Autodesk Fusion 360 part; units mm, degrees
(part 10 of 20)
  spline S928 degree 3 poles (18.9628, -686.0109) (18.8503, -686.0753) (18.6416, -686.1948) (18.4191, -686.286) (18.3165, -686.3281) knots 0 0 0 0 0.03884 0.072064 0.072064 0.072064 0.072064
  line L317 (18.3165, -686.3281) -> (18.3165, -685.7346)
  spline S929 degree 3 poles (18.3165, -685.7346) (18.4811, -685.6511) (18.8025, -685.4881) (19.081, -685.2595) (19.2169, -685.148) knots 0 0 0 0 0.05519 0.10775 0.10775 0.10775 0.10775
  spline S930 degree 3 poles (19.2169, -685.148) (19.3329, -685.0399) (19.5456, -684.8418) (19.6947, -684.5927) (19.7626, -684.4795) knots 0 0 0 0 0.047275 0.086674 0.086674 0.086674 0.086674
  line L318 (19.7626, -684.4795) -> (20.1582, -684.4795)
  line L319 (20.1582, -684.4795) -> (20.1583, -689.5)
  line L320 (29.2799, -739.4997) -> (29.2798, -735.8776)
  line L321 (29.2798, -735.8776) -> (29.8289, -735.8776)
  line L322 (29.8289, -735.8776) -> (29.8289, -736.3858)
  spline S931 degree 3 poles (29.8289, -736.3858) (29.8908, -736.3012) (30.0157, -736.1307) (30.1931, -736.0157) (30.2825, -735.9577) knots 0 0 0 0 0.031158 0.062835 0.062835 0.062835 0.062835
  spline S932 degree 3 poles (30.2825, -735.9577) (30.3817, -735.9105) (30.5856, -735.8134) (30.8112, -735.8017) (30.9271, -735.7957) knots 0 0 0 0 0.032617 0.067048 0.067048 0.067048 0.067048
  spline S933 degree 3 poles (30.9271, -735.7957) (31.0516, -735.8004) (31.284, -735.8093) (31.491, -735.9141) (31.5871, -735.9628) knots 0 0 0 0 0.036859 0.068796 0.068796 0.068796 0.068796
  spline S934 degree 3 poles (31.5871, -735.9628) (31.6668, -736.0245) (31.8277, -736.1492) (31.9092, -736.3358) (31.9503, -736.4301) knots 0 0 0 0 0.029725 0.060035 0.060035 0.060035 0.060035
  spline S935 degree 3 poles (31.9503, -736.4301) (32.1005, -736.2451) (32.3916, -735.8865) (32.848, -735.8253) (33.069, -735.7957) knots 0 0 0 0 0.068625 0.133023 0.133023 0.133023 0.133023
  spline S936 degree 3 poles (33.069, -735.7957) (33.2341, -735.8041) (33.542, -735.8197) (33.7851, -736.0072) (33.8978, -736.0941) knots 0 0 0 0 0.048244 0.08997 0.08997 0.08997 0.08997
  spline S937 degree 3 poles (33.8978, -736.0941) (33.9821, -736.2164) (34.1715, -736.4913) (34.1819, -736.8269) (34.1877, -737.0132) knots 0 0 0 0 0.043695 0.098195 0.098195 0.098195 0.098195
  line L323 (34.1877, -737.0132) -> (34.1878, -739.4996)
  line L324 (34.1878, -739.4996) -> (33.5773, -739.4996)
  line L325 (33.5773, -739.4996) -> (33.5772, -737.2179)
  spline S938 degree 3 poles (33.5772, -737.2179) (33.5772, -737.1117) (33.5772, -736.9323) (33.5348, -736.7584) (33.5175, -736.6875) knots 0 0 0 0 0.031711 0.053535 0.053535 0.053535 0.053535
  spline S939 degree 3 poles (33.5175, -736.6875) (33.4931, -736.6359) (33.4432, -736.5305) (33.349, -736.4617) (33.3009, -736.4266) knots 0 0 0 0 0.016863 0.034394 0.034394 0.034394 0.034394
  spline S940 degree 3 poles (33.3009, -736.4266) (33.2452, -736.3978) (33.1298, -736.338) (32.9998, -736.3312) (32.9326, -736.3277) knots 0 0 0 0 0.018597 0.038532 0.038532 0.038532 0.038532
  spline S941 degree 3 poles (32.9326, -736.3277) (32.8115, -736.3375) (32.5735, -736.3568) (32.3889, -736.5077) (32.2982, -736.5818) knots 0 0 0 0 0.035532 0.069798 0.069798 0.069798 0.069798
  spline S942 degree 3 poles (32.2982, -736.5818) (32.2249, -736.6885) (32.0578, -736.9317) (32.0501, -737.2286) (32.0459, -737.3953) knots 0 0 0 0 0.038079 0.086792 0.086792 0.086792 0.086792
  line L326 (32.0459, -737.3953) -> (32.0459, -739.4996)
  line L327 (32.0459, -739.4996) -> (31.432, -739.4997)
  line L328 (31.432, -739.4997) -> (31.4319, -737.1463)
  spline S943 degree 3 poles (31.4319, -737.1463) (31.4295, -737.0243) (31.4252, -736.8075) (31.3254, -736.6161) (31.2818, -736.5324) knots 0 0 0 0 0.036008 0.063954 0.063954 0.063954 0.063954
  spline S944 degree 3 poles (31.2818, -736.5324) (31.2196, -736.4728) (31.0834, -736.3424) (30.8937, -736.3329) (30.7907, -736.3278) knots 0 0 0 0 0.025037 0.054812 0.054812 0.054812 0.054812
  spline S945 degree 3 poles (30.7907, -736.3278) (30.706, -736.3335) (30.5365, -736.3448) (30.3865, -736.4244) (30.3115, -736.4642) knots 0 0 0 0 0.025172 0.050327 0.050327 0.050327 0.050327
  spline S946 degree 3 poles (30.3115, -736.4642) (30.2429, -736.5159) (30.1026, -736.6215) (30.0298, -736.7815) (29.9926, -736.8633) knots 0 0 0 0 0.025339 0.051812 0.051812 0.051812 0.051812
  spline S947 degree 3 poles (29.9926, -736.8633) (29.9639, -736.9696) (29.8971, -737.2171) (29.895, -737.4739) (29.8937, -737.6204) knots 0 0 0 0 0.032907 0.076633 0.076633 0.076633 0.076633
  line L329 (29.8937, -737.6204) -> (29.8938, -739.4997)
  line L330 (29.8938, -739.4997) -> (29.2799, -739.4997)
  line L331 (20.1598, -739.4999) -> (19.5459, -739.4999)
  line L332 (19.5459, -739.4999) -> (19.5458, -735.5879)
  spline S948 degree 3 poles (19.5458, -735.5879) (19.4621, -735.6608) (19.2807, -735.8186) (19.0751, -735.9436) (18.9643, -736.0109) knots 0 0 0 0 0.033221 0.072019 0.072019 0.072019 0.072019
  spline S949 degree 3 poles (18.9643, -736.0109) (18.8518, -736.0753) (18.6431, -736.1948) (18.4206, -736.286) (18.318, -736.3281) knots 0 0 0 0 0.03884 0.072064 0.072064 0.072064 0.072064
  line L333 (18.318, -736.3281) -> (18.318, -735.7346)
  spline S950 degree 3 poles (18.318, -735.7346) (18.4826, -735.6511) (18.804, -735.488) (19.0825, -735.2595) (19.2184, -735.148) knots 0 0 0 0 0.05519 0.10775 0.10775 0.10775 0.10775
  spline S951 degree 3 poles (19.2184, -735.148) (19.3344, -735.0399) (19.5471, -734.8418) (19.6962, -734.5927) (19.7641, -734.4795) knots 0 0 0 0 0.047275 0.086674 0.086674 0.086674 0.086674
  line L334 (19.7641, -734.4795) -> (20.1597, -734.4795)
  line L335 (20.1597, -734.4795) -> (20.1598, -739.4999)
  line L336 (28.5502, -789.465) -> (28.5499, -785.8429)
  line L337 (28.5499, -785.8429) -> (29.0991, -785.8429)
  line L338 (29.0991, -785.8429) -> (29.0991, -786.3511)
  spline S952 degree 3 poles (29.0991, -786.3511) (29.161, -786.2665) (29.2859, -786.096) (29.4633, -785.981) (29.5527, -785.923) knots 0 0 0 0 0.031158 0.062835 0.062835 0.062835 0.062835
  spline S953 degree 3 poles (29.5527, -785.923) (29.6519, -785.8758) (29.8557, -785.7786) (30.0814, -785.767) (30.1973, -785.761) knots 0 0 0 0 0.032617 0.067048 0.067048 0.067048 0.067048
  spline S954 degree 3 poles (30.1973, -785.761) (30.3218, -785.7657) (30.5542, -785.7745) (30.7612, -785.8794) (30.8572, -785.928) knots 0 0 0 0 0.036859 0.068796 0.068796 0.068796 0.068796
  spline S955 degree 3 poles (30.8572, -785.928) (30.9369, -785.9898) (31.0979, -786.1144) (31.1794, -786.301) (31.2205, -786.3953) knots 0 0 0 0 0.029725 0.060035 0.060035 0.060035 0.060035
  spline S956 degree 3 poles (31.2205, -786.3953) (31.3707, -786.2103) (31.6618, -785.8517) (32.1182, -785.7905) (32.3392, -785.7608) knots 0 0 0 0 0.068625 0.133023 0.133023 0.133023 0.133023
  spline S957 degree 3 poles (32.3392, -785.7608) (32.5042, -785.7692) (32.8121, -785.7849) (33.0552, -785.9723) (33.168, -786.0592) knots 0 0 0 0 0.048244 0.08997 0.08997 0.08997 0.08997
  spline S958 degree 3 poles (33.168, -786.0592) (33.2523, -786.1815) (33.4417, -786.4564) (33.4522, -786.792) (33.4579, -786.9783) knots 0 0 0 0 0.043695 0.098195 0.098195 0.098195 0.098195
  line L339 (33.4579, -786.9783) -> (33.4581, -789.4647)
  line L340 (33.4581, -789.4647) -> (32.8476, -789.4647)
  line L341 (32.8476, -789.4647) -> (32.8475, -787.183)
  spline S959 degree 3 poles (32.8475, -787.183) (32.8474, -787.0768) (32.8474, -786.8975) (32.805, -786.7235) (32.7877, -786.6526) knots 0 0 0 0 0.031711 0.053535 0.053535 0.053535 0.053535
  spline S960 degree 3 poles (32.7877, -786.6526) (32.7633, -786.601) (32.7134, -786.4956) (32.6192, -786.4268) (32.5711, -786.3918) knots 0 0 0 0 0.016863 0.034394 0.034394 0.034394 0.034394
  spline S961 degree 3 poles (32.5711, -786.3918) (32.5154, -786.3629) (32.4, -786.3032) (32.27, -786.2964) (32.2028, -786.2929) knots 0 0 0 0 0.018597 0.038532 0.038532 0.038532 0.038532
  spline S962 degree 3 poles (32.2028, -786.2929) (32.0816, -786.3027) (31.8437, -786.3219) (31.6591, -786.4729) (31.5684, -786.547) knots 0 0 0 0 0.035532 0.069798 0.069798 0.069798 0.069798
  spline S963 degree 3 poles (31.5684, -786.547) (31.4951, -786.6537) (31.328, -786.8969) (31.3204, -787.1938) (31.3161, -787.3605) knots 0 0 0 0 0.038079 0.086792 0.086792 0.086792 0.086792
  line L342 (31.3161, -787.3605) -> (31.3162, -789.4648)
  line L343 (31.3162, -789.4648) -> (30.7023, -789.4649)
  line L344 (30.7023, -789.4649) -> (30.7022, -787.1115)
  spline S964 degree 3 poles (30.7022, -787.1115) (30.6997, -786.9895) (30.6954, -786.7727) (30.5956, -786.5813) (30.552, -786.4976) knots 0 0 0 0 0.036008 0.063954 0.063954 0.063954 0.063954
  spline S965 degree 3 poles (30.552, -786.4976) (30.4898, -786.4381) (30.3536, -786.3077) (30.1639, -786.2982) (30.0609, -786.293) knots 0 0 0 0 0.025037 0.054812 0.054812 0.054812 0.054812
  spline S966 degree 3 poles (30.0609, -786.293) (29.9761, -786.2987) (29.8067, -786.3101) (29.6567, -786.3897) (29.5817, -786.4295) knots 0 0 0 0 0.025172 0.050327 0.050327 0.050327 0.050327
  spline S967 degree 3 poles (29.5817, -786.4295) (29.5131, -786.4812) (29.3728, -786.5868) (29.3, -786.7468) (29.2628, -786.8286) knots 0 0 0 0 0.025339 0.051812 0.051812 0.051812 0.051812
  spline S968 degree 3 poles (29.2628, -786.8286) (29.2341, -786.9349) (29.1673, -787.1824) (29.1652, -787.4392) (29.164, -787.5857) knots 0 0 0 0 0.032907 0.076633 0.076633 0.076633 0.076633
  line L345 (29.164, -787.5857) -> (29.1641, -789.465)
  line L346 (29.1641, -789.465) -> (28.5502, -789.465)
  line L347 (27.416, -838.1729) -> (28.0197, -838.2513)
  spline S969 degree 3 poles (28.0197, -838.2513) (27.9771, -838.4452) (27.8953, -838.817) (27.6369, -839.0953) (27.5133, -839.2285) knots 0 0 0 0 0.058356 0.111856 0.111856 0.111856 0.111856
  spline S970 degree 3 poles (27.5133, -839.2285) (27.3672, -839.3314) (27.0671, -839.5429) (26.7004, -839.5684) (26.5123, -839.5815) knots 0 0 0 0 0.052559 0.107965 0.107965 0.107965 0.107965
  spline S971 degree 3 poles (26.5123, -839.5815) (26.2792, -839.564) (25.8276, -839.5301) (25.4834, -839.2373) (25.3168, -839.0956) knots 0 0 0 0 0.068154 0.132052 0.132052 0.132052 0.132052
  spline S972 degree 3 poles (25.3168, -839.0956) (25.1853, -838.9048) (24.8974, -838.4874) (24.8763, -837.9786) (24.8649, -837.7023) knots 0 0 0 0 0.068157 0.149141 0.149141 0.149141 0.149141
  spline S973 degree 3 poles (24.8649, -837.7023) (24.8712, -837.5171) (24.8832, -837.1646) (25.0026, -836.833) (25.0592, -836.6757) knots 0 0 0 0 0.055211 0.105055 0.105055 0.105055 0.105055
  spline S974 degree 3 poles (25.0592, -836.6757) (25.1314, -836.5388) (25.2736, -836.2692) (25.5265, -836.0993) (25.651, -836.0157) knots 0 0 0 0 0.04564 0.089884 0.089884 0.089884 0.089884
  spline S975 degree 3 poles (25.651, -836.0157) (25.7869, -835.9516) (26.0608, -835.8223) (26.3632, -835.8046) (26.5156, -835.7957) knots 0 0 0 0 0.044643 0.089955 0.089955 0.089955 0.089955
  spline S976 degree 3 poles (26.5156, -835.7957) (26.6993, -835.8051) (27.0472, -835.8228) (27.3418, -836.0071) (27.4808, -836.0941) knots 0 0 0 0 0.054149 0.102527 0.102527 0.102527 0.102527
  spline S977 degree 3 poles (27.4808, -836.0941) (27.5953, -836.2076) (27.8343, -836.4446) (27.9181, -836.7714) (27.9617, -836.9416) knots 0 0 0 0 0.047449 0.099081 0.099081 0.099081 0.099081
  line L348 (27.9617, -836.9416) -> (27.3648, -837.0337)
  spline S978 degree 3 poles (27.3648, -837.0337) (27.334, -836.9224) (27.2765, -836.7149) (27.1306, -836.5575) (27.063, -836.4846) knots 0 0 0 0 0.034086 0.063475 0.063475 0.063475 0.063475
  spline S979 degree 3 poles (27.063, -836.4846) (26.986, -836.4309) (26.8287, -836.3212) (26.6372, -836.3075) (26.5394, -836.3005) knots 0 0 0 0 0.027619 0.056426 0.056426 0.056426 0.056426
  spline S980 degree 3 poles (26.5394, -836.3005) (26.3928, -836.3135) (26.1037, -836.3393) (25.8907, -836.5361) (25.7857, -836.6331) knots 0 0 0 0 0.04285 0.084486 0.084486 0.084486 0.084486
  spline S981 degree 3 poles (25.7857, -836.6331) (25.7015, -836.7726) (25.5077, -837.0941) (25.5001, -837.4716) (25.4958, -837.6852) knots 0 0 0 0 0.048123 0.11083 0.11083 0.11083 0.11083
  spline S982 degree 3 poles (25.4958, -837.6852) (25.4994, -837.901) (25.5057, -838.2797) (25.6944, -838.6057) (25.7755, -838.7459) knots 0 0 0 0 0.063398 0.111295 0.111295 0.111295 0.111295
  spline S983 degree 3 poles (25.7755, -838.7459) (25.8767, -838.8424) (26.0813, -839.0376) (26.363, -839.0636) (26.5054, -839.0768) knots 0 0 0 0 0.040675 0.082263 0.082263 0.082263 0.082263
  spline S984 degree 3 poles (26.5054, -839.0768) (26.6198, -839.0685) (26.8427, -839.0525) (27.0219, -838.9197) (27.1091, -838.855) knots 0 0 0 0 0.033628 0.065508 0.065508 0.065508 0.065508
  spline S985 degree 3 poles (27.1091, -838.855) (27.1832, -838.7651) (27.3466, -838.5664) (27.3915, -838.312) (27.416, -838.1729) knots 0 0 0 0 0.034396 0.07593 0.07593 0.07593 0.07593
  spline S986 degree 3 poles (19.0565, -837.034) (19.0601, -836.7657) (19.0666, -836.2825) (19.1859, -835.8147) (19.2389, -835.6067) knots 0 0 0 0 0.080152 0.144341 0.144341 0.144341 0.144341
  spline S987 degree 3 poles (19.2389, -835.6067) (19.3036, -835.4398) (19.4261, -835.1233) (19.6672, -834.8853) (19.7812, -834.7728) knots 0 0 0 0 0.052977 0.10048 0.10048 0.10048 0.10048
  spline S988 degree 3 poles (19.7812, -834.7728) (19.9126, -834.6872) (20.1874, -834.5083) (20.5155, -834.4893) (20.6867, -834.4794) knots 0 0 0 0 0.046203 0.096661 0.096661 0.096661 0.096661
  spline S989 degree 3 poles (20.6867, -834.4794) (20.8145, -834.485) (21.06, -834.4957) (21.2849, -834.5942) (21.3927, -834.6414) knots 0 0 0 0 0.037989 0.072993 0.072993 0.072993 0.072993
  spline S990 degree 3 poles (21.3927, -834.6414) (21.49, -834.7021) (21.6873, -834.8253) (21.8245, -835.0133) (21.8941, -835.1086) knots 0 0 0 0 0.034048 0.069103 0.069103 0.069103 0.069103
  spline S991 degree 3 poles (21.8941, -835.1086) (21.9574, -835.2196) (22.0914, -835.4545) (22.1655, -835.7148) (22.2045, -835.8521) knots 0 0 0 0 0.038176 0.080832 0.080832 0.080832 0.080832
  spline S992 degree 3 poles (22.2045, -835.8521) (22.2372, -836.0232) (22.3118, -836.4133) (22.3152, -836.8108) (22.3171, -837.0339) knots 0 0 0 0 0.052146 0.118926 0.118926 0.118926 0.118926
  spline S993 degree 3 poles (22.3171, -837.0339) (22.3135, -837.3005) (22.3069, -837.7813) (22.1889, -838.247) (22.1364, -838.4545) knots 0 0 0 0 0.079639 0.143634 0.143634 0.143634 0.143634
  spline S994 degree 3 poles (22.1364, -838.4545) (22.0722, -838.6214) (21.9504, -838.9384) (21.7097, -839.1771) (21.5958, -839.2901) knots 0 0 0 0 0.052961 0.100531 0.100531 0.100531 0.100531
  spline S995 degree 3 poles (21.5958, -839.2901) (21.4642, -839.3761) (21.1885, -839.5562) (20.8591, -839.5752) (20.6869, -839.5851) knots 0 0 0 0 0.046339 0.097057 0.097057 0.097057 0.097057
  spline S996 degree 3 poles (20.6869, -839.5851) (20.4607, -839.5658) (20.0194, -839.5282) (19.7046, -839.2179) (19.5511, -839.0668) knots 0 0 0 0 0.065835 0.128409 0.128409 0.128409 0.128409
  spline S997 degree 3 poles (19.5511, -839.0668) (19.4077, -838.7987) (19.0701, -838.1677) (19.0615, -837.448) (19.0565, -837.034) knots 0 0 0 0 0.090022 0.211899 0.211899 0.211899 0.211899
  line L349 (5, 0) -> (5, -3)
  line L350 (5, -3) -> (0, -3)
  line L351 (0, -3) -> (0, -36.5)
  line L352 (0, -36.5) -> (17.5, -36.5)
  line L353 (17.5, -36.5) -> (17.5, -37.5)
  line L354 (17.5, -37.5) -> (0, -37.5)
  line L355 (0, -37.5) -> (0, -46.5)
  line L356 (0, -46.5) -> (17.5, -46.5)
  line L357 (17.5, -46.5) -> (17.5, -47.5)
  line L358 (17.5, -47.5) -> (0, -47.5)
  line L359 (0, -47.5) -> (0, -56.5)
  line L360 (0, -56.5) -> (17.5, -56.5)
  line L361 (17.5, -56.5) -> (17.5, -57.5)
  line L362 (17.5, -57.5) -> (0, -57.5)
  line L363 (0, -57.5) -> (0, -66.5)
  line L364 (0, -66.5) -> (17.5, -66.5)
  line L365 (17.5, -66.5) -> (17.5, -67.5)
  line L366 (17.5, -67.5) -> (0, -67.5)
  line L367 (0, -67.5) -> (0, -76.5)
  line L368 (0, -76.5) -> (17.5, -76.5)
  line L369 (17.5, -76.5) -> (17.5, -77.5)
  line L370 (17.5, -77.5) -> (0, -77.5)
  line L371 (0, -77.5) -> (0, -86.5)
  line L372 (0, -86.5) -> (17.5, -86.5)
  line L373 (17.5, -86.5) -> (17.5, -87.5)
  line L374 (17.5, -87.5) -> (0, -87.5)
  line L375 (0, -87.5) -> (0, -96.5)
  line L376 (0, -96.5) -> (17.5, -96.5)
  line L377 (17.5, -96.5) -> (17.5, -97.5)
  line L378 (17.5, -97.5) -> (0, -97.5)
  line L379 (0, -97.5) -> (0, -106.5)
  line L380 (0, -106.5) -> (17.5, -106.5)
  line L381 (17.5, -106.5) -> (17.5, -107.5)
  line L382 (17.5, -107.5) -> (0, -107.5)
  line L383 (0, -107.5) -> (0, -116.5)
  line L384 (0, -116.5) -> (17.5, -116.5)
  line L385 (17.5, -116.5) -> (17.5, -117.5)
  line L386 (17.5, -117.5) -> (0, -117.5)
  line L387 (0, -117.5) -> (0, -126.5)
  line L388 (0, -126.5) -> (17.5, -126.5)
  line L389 (17.5, -126.5) -> (17.5, -127.5)
  line L390 (17.5, -127.5) -> (0, -127.5)
  line L391 (0, -127.5) -> (0, -136.5)
  line L392 (0, -136.5) -> (17.5, -136.5)
  line L393 (17.5, -136.5) -> (17.5, -137.5)
  line L394 (17.5, -137.5) -> (0, -137.5)
  line L395 (0, -137.5) -> (0, -146.5)
  line L396 (0, -146.5) -> (17.5, -146.5)
  line L397 (17.5, -146.5) -> (17.5, -147.5)
  line L398 (17.5, -147.5) -> (0, -147.5)
  line L399 (0, -147.5) -> (0, -156.5)
  line L400 (0, -156.5) -> (17.5, -156.5)
  line L401 (17.5, -156.5) -> (17.5, -157.5)
  line L402 (17.5, -157.5) -> (0, -157.5)
  line L403 (0, -157.5) -> (0, -166.5)
  line L404 (0, -166.5) -> (17.5, -166.5)
  line L405 (17.5, -166.5) -> (17.5, -167.5)
  line L406 (17.5, -167.5) -> (0, -167.5)
  line L407 (0, -167.5) -> (0, -176.5)
  line L408 (0, -176.5) -> (17.5, -176.5)
  line L409 (17.5, -176.5) -> (17.5, -177.5)
  line L410 (17.5, -177.5) -> (0, -177.5)
  line L411 (0, -177.5) -> (0, -186.5)
  line L412 (0, -186.5) -> (17.5, -186.5)
  line L413 (17.5, -186.5) -> (17.5, -187.5)
  line L414 (17.5, -187.5) -> (0, -187.5)
  line L415 (0, -187.5) -> (0, -196.5)
  line L416 (0, -196.5) -> (17.5, -196.5)
  line L417 (17.5, -196.5) -> (17.5, -197.5)
  line L418 (17.5, -197.5) -> (0, -197.5)
  line L419 (0, -197.5) -> (0, -206.5)
  line L420 (0, -206.5) -> (17.5, -206.5)
  line L421 (17.5, -206.5) -> (17.5, -207.5)
  line L422 (17.5, -207.5) -> (0, -207.5)
  line L423 (0, -207.5) -> (0, -216.5)
  line L424 (0, -216.5) -> (17.5, -216.5)
  line L425 (17.5, -216.5) -> (17.5, -217.5)
  line L426 (17.5, -217.5) -> (0, -217.5)
  line L427 (0, -217.5) -> (0, -226.5)
  line L428 (0, -226.5) -> (17.5, -226.5)
  line L429 (17.5, -226.5) -> (17.5, -227.5)
  line L430 (17.5, -227.5) -> (0, -227.5)
  line L431 (0, -227.5) -> (0, -236.5)
  line L432 (0, -236.5) -> (17.5, -236.5)
  line L433 (17.5, -236.5) -> (17.5, -237.5)
  line L434 (17.5, -237.5) -> (0, -237.5)
  line L435 (0, -237.5) -> (0, -246.5)
  line L436 (0, -246.5) -> (17.5, -246.5)
  line L437 (17.5, -246.5) -> (17.5, -247.5)
  line L438 (17.5, -247.5) -> (0, -247.5)
  line L439 (0, -247.5) -> (0, -256.5)
  line L440 (0, -256.5) -> (17.5, -256.5)
  line L441 (17.5, -256.5) -> (17.5, -257.5)
  line L442 (17.5, -257.5) -> (0, -257.5)
  line L443 (0, -257.5) -> (0, -266.5)
  line L444 (0, -266.5) -> (17.5, -266.5)
  line L445 (17.5, -266.5) -> (17.5, -267.5)
  line L446 (17.5, -267.5) -> (0, -267.5)
  line L447 (0, -267.5) -> (0, -276.5)
  line L448 (0, -276.5) -> (17.5, -276.5)
  line L449 (17.5, -276.5) -> (17.5, -277.5)
  line L450 (17.5, -277.5) -> (0, -277.5)
  line L451 (0, -277.5) -> (0, -286.5)
  line L452 (0, -286.5) -> (17.5, -286.5)
  line L453 (17.5, -286.5) -> (17.5, -287.5)
  line L454 (17.5, -287.5) -> (0, -287.5)
  line L455 (0, -287.5) -> (0, -296.5)
  line L456 (0, -296.5) -> (17.5, -296.5)
  line L457 (17.5, -296.5) -> (17.5, -297.5)
  line L458 (17.5, -297.5) -> (0, -297.5)
  line L459 (0, -297.5) -> (0, -306.5)
  line L460 (0, -306.5) -> (17.5, -306.5)
  line L461 (17.5, -306.5) -> (17.5, -307.5)
  line L462 (17.5, -307.5) -> (0, -307.5)
  line L463 (0, -307.5) -> (0, -316.5)
  line L464 (0, -316.5) -> (17.5, -316.5)
  line L465 (17.5, -316.5) -> (17.5, -317.5)
  line L466 (17.5, -317.5) -> (0, -317.5)
  line L467 (0, -317.5) -> (0, -326.5)
  line L468 (0, -326.5) -> (17.5, -326.5)
  line L469 (17.5, -326.5) -> (17.5, -327.5)
  line L470 (17.5, -327.5) -> (0, -327.5)
  line L471 (0, -327.5) -> (0, -336.5)
  line L472 (0, -336.5) -> (17.5, -336.5)
  line L473 (17.5, -336.5) -> (17.5, -337.5)
  line L474 (17.5, -337.5) -> (0, -337.5)
  line L475 (0, -337.5) -> (0, -346.5)
  line L476 (0, -346.5) -> (17.5, -346.5)
  line L477 (17.5, -346.5) -> (17.5, -347.5)
  line L478 (17.5, -347.5) -> (0, -347.5)
  line L479 (0, -347.5) -> (0, -356.5)
  line L480 (0, -356.5) -> (17.5, -356.5)
  line L481 (17.5, -356.5) -> (17.5, -357.5)
  line L482 (17.5, -357.5) -> (0, -357.5)
  line L483 (0, -357.5) -> (0, -366.5)
  line L484 (0, -366.5) -> (17.5, -366.5)
  line L485 (17.5, -366.5) -> (17.5, -367.5)
  line L486 (17.5, -367.5) -> (0, -367.5)
  line L487 (0, -367.5) -> (0, -376.5)
  line L488 (0, -376.5) -> (17.5, -376.5)
  line L489 (17.5, -376.5) -> (17.5, -377.5)
  line L490 (17.5, -377.5) -> (0, -377.5)
  line L491 (0, -377.5) -> (0, -386.5)
  line L492 (0, -386.5) -> (17.5, -386.5)
  line L493 (17.5, -386.5) -> (17.5, -387.5)
  line L494 (17.5, -387.5) -> (0, -387.5)
  line L495 (0, -387.5) -> (0, -396.5)
  line L496 (0, -396.5) -> (17.5, -396.5)
  line L497 (17.5, -396.5) -> (17.5, -397.5)
  line L498 (17.5, -397.5) -> (0, -397.5)
  line L499 (0, -397.5) -> (0, -406.5)
  line L500 (0, -406.5) -> (17.5, -406.5)
  line L501 (17.5, -406.5) -> (17.5, -407.5)
  line L502 (17.5, -407.5) -> (0, -407.5)
  line L503 (0, -407.5) -> (0, -416.5)
  line L504 (0, -416.5) -> (17.5, -416.5)
  line L505 (17.5, -416.5) -> (17.5, -417.5)
  line L506 (17.5, -417.5) -> (0, -417.5)
  line L507 (0, -417.5) -> (0, -426.5)
  line L508 (0, -426.5) -> (17.5, -426.5)
  line L509 (17.5, -426.5) -> (17.5, -427.5)
  line L510 (17.5, -427.5) -> (0, -427.5)
  line L511 (0, -427.5) -> (0, -436.5)
  line L512 (0, -436.5) -> (17.5, -436.5)
  line L513 (17.5, -436.5) -> (17.5, -437.5)
  line L514 (17.5, -437.5) -> (0, -437.5)
  line L515 (0, -437.5) -> (0, -446.5)
  line L516 (0, -446.5) -> (17.5, -446.5)
  line L517 (17.5, -446.5) -> (17.5, -447.5)
  line L518 (17.5, -447.5) -> (0, -447.5)
  line L519 (0, -447.5) -> (0, -456.5)
  line L520 (0, -456.5) -> (17.5, -456.5)
  line L521 (17.5, -456.5) -> (17.5, -457.5)
  line L522 (17.5, -457.5) -> (0, -457.5)
  line L523 (0, -457.5) -> (0, -466.5)
  line L524 (0, -466.5) -> (17.5, -466.5)
  line L525 (17.5, -466.5) -> (17.5, -467.5)
  line L526 (17.5, -467.5) -> (0, -467.5)
  line L527 (0, -467.5) -> (0, -476.5)
  line L528 (0, -476.5) -> (17.5, -476.5)
  line L529 (17.5, -476.5) -> (17.5, -477.5)
  line L530 (17.5, -477.5) -> (0, -477.5)
  line L531 (0, -477.5) -> (0, -486.5)
  line L532 (0, -486.5) -> (17.5, -486.5)
  line L533 (17.5, -486.5) -> (17.5, -487.5)
  line L534 (17.5, -487.5) -> (0, -487.5)
  line L535 (0, -487.5) -> (0, -496.5)
  line L536 (0, -496.5) -> (17.5, -496.5)
  line L537 (17.5, -496.5) -> (17.5, -497.5)
  line L538 (17.5, -497.5) -> (0, -497.5)
  line L539 (0, -497.5) -> (0, -506.5)
  line L540 (0, -506.5) -> (17.5, -506.5)
  line L541 (17.5, -506.5) -> (17.5, -507.5)
  line L542 (17.5, -507.5) -> (0, -507.5)
  line L543 (0, -507.5) -> (0, -516.5)
  line L544 (0, -516.5) -> (17.5, -516.5)
  line L545 (17.5, -516.5) -> (17.5, -517.5)
  line L546 (17.5, -517.5) -> (0, -517.5)
  line L547 (0, -517.5) -> (0, -526.5)
  line L548 (0, -526.5) -> (17.5, -526.5)
  line L549 (17.5, -526.5) -> (17.5, -527.5)
  line L550 (17.5, -527.5) -> (0, -527.5)
  line L551 (0, -527.5) -> (0, -536.5)
  line L552 (0, -536.5) -> (17.5, -536.5)
  line L553 (17.5, -536.5) -> (17.5, -537.5)
  line L554 (17.5, -537.5) -> (0, -537.5)
  line L555 (0, -537.5) -> (0, -546.5)
  line L556 (0, -546.5) -> (17.5, -546.5)
  line L557 (17.5, -546.5) -> (17.5, -547.5)
  line L558 (17.5, -547.5) -> (0, -547.5)
  line L559 (0, -547.5) -> (0, -556.5)
  line L560 (0, -556.5) -> (17.5, -556.5)
  line L561 (17.5, -556.5) -> (17.5, -557.5)
  line L562 (17.5, -557.5) -> (0, -557.5)
  line L563 (0, -557.5) -> (0, -566.5)
  line L564 (0, -566.5) -> (17.5, -566.5)
  line L565 (17.5, -566.5) -> (17.5, -567.5)
  line L566 (17.5, -567.5) -> (0, -567.5)
  line L567 (0, -567.5) -> (0, -576.5)
  line L568 (0, -576.5) -> (17.5, -576.5)
  line L569 (17.5, -576.5) -> (17.5, -577.5)
  line L570 (17.5, -577.5) -> (0, -577.5)
  line L571 (0, -577.5) -> (0, -586.5)
  line L572 (0, -586.5) -> (17.5, -586.5)
  line L573 (17.5, -586.5) -> (17.5, -587.5)
  line L574 (17.5, -587.5) -> (0, -587.5)
  line L575 (0, -587.5) -> (0, -596.5)
  line L576 (0, -596.5) -> (17.5, -596.5)
  line L577 (17.5, -596.5) -> (17.5, -597.5)
  line L578 (17.5, -597.5) -> (0, -597.5)
  line L579 (0, -597.5) -> (0, -606.5)
  line L580 (0, -606.5) -> (17.5, -606.5)
  line L581 (17.5, -606.5) -> (17.5, -607.5)
  line L582 (17.5, -607.5) -> (0, -607.5)
  line L583 (0, -607.5) -> (0, -616.5)
  line L584 (0, -616.5) -> (17.5, -616.5)
  line L585 (17.5, -616.5) -> (17.5, -617.5)
  line L586 (17.5, -617.5) -> (0, -617.5)
  line L587 (0, -617.5) -> (0, -626.5)
  line L588 (0, -626.5) -> (17.5, -626.5)
  line L589 (17.5, -626.5) -> (17.5, -627.5)
  line L590 (17.5, -627.5) -> (0, -627.5)
  line L591 (0, -627.5) -> (0, -636.5)
  line L592 (0, -636.5) -> (17.5, -636.5)
  line L593 (17.5, -636.5) -> (17.5, -637.5)
  line L594 (17.5, -637.5) -> (0, -637.5)
  line L595 (0, -637.5) -> (0, -646.5)
  line L596 (0, -646.5) -> (17.5, -646.5)
  line L597 (17.5, -646.5) -> (17.5, -647.5)
  line L598 (17.5, -647.5) -> (0, -647.5)
  line L599 (0, -647.5) -> (0, -656.5)
  line L600 (0, -656.5) -> (17.5, -656.5)
  line L601 (17.5, -656.5) -> (17.5, -657.5)
  line L602 (17.5, -657.5) -> (0, -657.5)
  line L603 (0, -657.5) -> (0, -666.5)
  line L604 (0, -666.5) -> (17.5, -666.5)
  line L605 (17.5, -666.5) -> (17.5, -667.5)
  line L606 (17.5, -667.5) -> (0, -667.5)
  line L607 (0, -667.5) -> (0, -676.5)
  line L608 (0, -676.5) -> (17.5, -676.5)
  line L609 (17.5, -676.5) -> (17.5, -677.5)
  line L610 (17.5, -677.5) -> (0, -677.5)
  line L611 (0, -677.5) -> (0, -686.5)
  line L612 (0, -686.5) -> (17.5, -686.5)
  line L613 (17.5, -686.5) -> (17.5, -687.5)
  line L614 (17.5, -687.5) -> (0, -687.5)
  line L615 (0, -687.5) -> (0, -696.5)
  line L616 (0, -696.5) -> (17.5, -696.5)
  line L617 (17.5, -696.5) -> (17.5, -697.5)
  line L618 (17.5, -697.5) -> (0, -697.5)
  line L619 (0, -697.5) -> (0, -706.5)
  line L620 (0, -706.5) -> (17.5, -706.5)
  line L621 (17.5, -706.5) -> (17.5, -707.5)
  line L622 (17.5, -707.5) -> (0, -707.5)
  line L623 (0, -707.5) -> (0, -716.5)
  line L624 (0, -716.5) -> (17.5, -716.5)
  line L625 (17.5, -716.5) -> (17.5, -717.5)
  line L626 (17.5, -717.5) -> (0, -717.5)
  line L627 (0, -717.5) -> (0, -726.5)
  line L628 (0, -726.5) -> (17.5, -726.5)
  line L629 (17.5, -726.5) -> (17.5, -727.5)
  line L630 (17.5, -727.5) -> (0, -727.5)
  line L631 (0, -727.5) -> (0, -736.5)
  line L632 (0, -736.5) -> (17.5, -736.5)
  line L633 (17.5, -736.5) -> (17.5, -737.5)
  line L634 (17.5, -737.5) -> (0, -737.5)
  line L635 (0, -737.5) -> (0, -746.5)
  line L636 (0, -746.5) -> (17.5, -746.5)
  line L637 (17.5, -746.5) -> (17.5, -747.5)
  line L638 (17.5, -747.5) -> (0, -747.5)
  line L639 (0, -747.5) -> (0, -756.5)
  line L640 (0, -756.5) -> (17.5, -756.5)
  line L641 (17.5, -756.5) -> (17.5, -757.5)
  line L642 (17.5, -757.5) -> (0, -757.5)
  line L643 (0, -757.5) -> (0, -766.5)
  line L644 (0, -766.5) -> (17.5, -766.5)
  line L645 (17.5, -766.5) -> (17.5, -767.5)
  line L646 (17.5, -767.5) -> (0, -767.5)
  line L647 (0, -767.5) -> (0, -776.5)
  line L648 (0, -776.5) -> (17.5, -776.5)
  line L649 (17.5, -776.5) -> (17.5, -777.5)
  line L650 (17.5, -777.5) -> (0, -777.5)
  line L651 (0, -777.5) -> (0, -786.5)
  line L652 (0, -786.5) -> (17.5, -786.5)
  line L653 (17.5, -786.5) -> (17.5, -787.5)
  line L654 (17.5, -787.5) -> (0, -787.5)
  line L655 (0, -787.5) -> (0, -796.5)
  line L656 (0, -796.5) -> (17.5, -796.5)
  line L657 (17.5, -796.5) -> (17.5, -797.5)
  line L658 (17.5, -797.5) -> (0, -797.5)
  line L659 (0, -797.5) -> (0, -806.5)
  line L660 (0, -806.5) -> (17.5, -806.5)
  line L661 (17.5, -806.5) -> (17.5, -807.5)
  line L662 (17.5, -807.5) -> (0, -807.5)
  line L663 (0, -807.5) -> (0, -816.5)
  line L664 (0, -816.5) -> (17.5, -816.5)
  line L665 (17.5, -816.5) -> (17.5, -817.5)
  line L666 (17.5, -817.5) -> (0, -817.5)
  line L667 (0, -817.5) -> (0, -826.5)
  line L668 (0, -826.5) -> (17.5, -826.5)
  line L669 (17.5, -826.5) -> (17.5, -827.5)
  line L670 (17.5, -827.5) -> (0, -827.5)
  line L671 (0, -827.5) -> (0, -836.5)
  line L672 (0, -836.5) -> (17.5, -836.5)
  line L673 (17.5, -836.5) -> (17.5, -837.5)
  line L674 (17.5, -837.5) -> (0, -837.5)
  line L675 (0, -837.5) -> (0, -870.7)
  line L676 (0, -870.7) -> (5, -870.7)
  line L677 (5, -870.7) -> (5, -874)
  line L678 (5, -874) -> (35, -874)
  line L679 (35, -874) -> (35, -870.7)
  line L680 (35, -870.7) -> (40, -870.7)
  line L681 (40, -870.7) -> (40, -3)
  line L682 (40, -3) -> (35, -3)
  line L683 (35, -3) -> (35, 0)
  line L684 (35, 0) -> (5, 0)
  spline S998 degree 3 poles (22.5989, -37.0341) (22.5954, -37.3816) (22.5897, -37.949) (22.804, -38.4707) (22.8871, -38.6729) knots 0 0 0 0 0.102785 0.167831 0.167831 0.167831 0.167831
  spline S999 degree 3 poles (22.8871, -38.6729) (22.985, -38.7917) (23.1716, -39.0182) (23.4607, -39.0604) (23.5982, -39.0805) knots 0 0 0 0 0.04439 0.084625 0.084625 0.084625 0.084625
  spline S1000 degree 3 poles (23.5982, -39.0805) (23.7357, -39.0603) (24.0252, -39.0177) (24.2115, -38.7905) (24.3093, -38.6712) knots 0 0 0 0 0.040246 0.084724 0.084724 0.084724 0.084724
  spline S1001 degree 3 poles (24.3093, -38.6712) (24.3924, -38.4689) (24.6064, -37.9476) (24.6009, -37.3809) (24.5975, -37.0341) knots 0 0 0 0 0.065086 0.167658 0.167658 0.167658 0.167658
  spline S1002 degree 3 poles (24.5975, -37.0341) (24.6012, -36.6859) (24.6071, -36.1179) (24.3924, -35.5957) (24.3093, -35.3936) knots 0 0 0 0 0.102998 0.168003 0.168003 0.168003 0.168003
  spline S1003 degree 3 poles (24.3093, -35.3936) (24.2108, -35.2753) (24.0218, -35.0485) (23.7306, -35.0074) (23.5914, -34.9877) knots 0 0 0 0 0.044426 0.085146 0.085146 0.085146 0.085146
  spline S1004 degree 3 poles (23.5914, -34.9877) (23.4571, -35.0033) (23.1857, -35.0347) (23.0066, -35.2414) (22.9161, -35.3458) knots 0 0 0 0 0.039068 0.078965 0.078965 0.078965 0.078965
  spline S1005 degree 3 poles (22.9161, -35.3458) (22.8245, -35.56) (22.5952, -36.096) (22.5975, -36.6822) (22.5989, -37.0341) knots 0 0 0 0 0.069271 0.173342 0.173342 0.173342 0.173342
  spline S1006 degree 3 poles (18.9052, -35.7483) (18.9136, -35.86) (18.9299, -36.0773) (19.0671, -36.2461) (19.1337, -36.3281) knots 0 0 0 0 0.032733 0.063665 0.063665 0.063665 0.063665
  spline S1007 degree 3 poles (19.1337, -36.3281) (19.2176, -36.3937) (19.3917, -36.5299) (19.6127, -36.5453) (19.7271, -36.5532) knots 0 0 0 0 0.03122 0.064779 0.064779 0.064779 0.064779
  spline S1008 degree 3 poles (19.7271, -36.5532) (19.8388, -36.5451) (20.0556, -36.5293) (20.226, -36.395) (20.3087, -36.3298) knots 0 0 0 0 0.032753 0.063582 0.063582 0.063582 0.063582
  spline S1009 degree 3 poles (20.3087, -36.3298) (20.3748, -36.2509) (20.5078, -36.0923) (20.5262, -35.886) (20.5355, -35.7824) knots 0 0 0 0 0.030119 0.060538 0.060538 0.060538 0.060538
  spline S1010 degree 3 poles (20.5355, -35.7824) (20.5261, -35.6746) (20.5074, -35.4609) (20.37, -35.2962) (20.3018, -35.2145) knots 0 0 0 0 0.031624 0.062735 0.062735 0.062735 0.062735
  spline S1011 degree 3 poles (20.3018, -35.2145) (20.2183, -35.1474) (20.0483, -35.0109) (19.8309, -34.9933) (19.7203, -34.9843) knots 0 0 0 0 0.031394 0.063841 0.063841 0.063841 0.063841
  spline S1012 degree 3 poles (19.7203, -34.9843) (19.6091, -34.9928) (19.3919, -35.0093) (19.2207, -35.1438) (19.1371, -35.2094) knots 0 0 0 0 0.032634 0.063783 0.063783 0.063783 0.063783
  spline S1013 degree 3 poles (19.1371, -35.2094) (19.0695, -35.2877) (18.9353, -35.443) (18.9152, -35.6471) (18.9052, -35.7483) knots 0 0 0 0 0.030232 0.059964 0.059964 0.059964 0.059964
  spline S1014 degree 3 poles (18.7074, -38.0573) (18.7128, -38.1446) (18.7238, -38.3214) (18.7955, -38.4835) (18.8318, -38.5655) knots 0 0 0 0 0.026022 0.052693 0.052693 0.052693 0.052693
  spline S1015 degree 3 poles (18.8318, -38.5655) (18.8786, -38.6428) (18.9725, -38.7982) (19.1252, -38.8964) (19.2019, -38.9458) knots 0 0 0 0 0.026723 0.053693 0.053693 0.053693 0.053693
  spline S1016 degree 3 poles (19.2019, -38.9458) (19.2854, -38.9851) (19.453, -39.0639) (19.6379, -39.0749) (19.7305, -39.0805) knots 0 0 0 0 0.027424 0.055001 0.055001 0.055001 0.055001
  spline S1017 degree 3 poles (19.7305, -39.0805) (19.8696, -39.0699) (20.1409, -39.0493) (20.3534, -38.88) (20.457, -38.7974) knots 0 0 0 0 0.040779 0.079588 0.079588 0.079588 0.079588
  spline S1018 degree 3 poles (20.457, -38.7974) (20.5406, -38.6951) (20.7115, -38.4857) (20.7327, -38.2158) (20.7435, -38.0778) knots 0 0 0 0 0.038665 0.079124 0.079124 0.079124 0.079124
  spline S1019 degree 3 poles (20.7435, -38.0778) (20.7322, -37.9374) (20.71, -37.6619) (20.5345, -37.4489) (20.4485, -37.3445) knots 0 0 0 0 0.041167 0.080756 0.080756 0.080756 0.080756
  spline S1020 degree 3 poles (20.4485, -37.3445) (20.3426, -37.2599) (20.1266, -37.0875) (19.8507, -37.0657) (19.7101, -37.0546) knots 0 0 0 0 0.039695 0.080966 0.080966 0.080966 0.080966
  spline S1021 degree 3 poles (19.7101, -37.0546) (19.5729, -37.0655) (19.3037, -37.0871) (19.0946, -37.2575) (18.9921, -37.3411) knots 0 0 0 0 0.040248 0.078949 0.078949 0.078949 0.078949
  spline S1022 degree 3 poles (18.9921, -37.3411) (18.9091, -37.4437) (18.74, -37.6527) (18.7184, -37.9209) (18.7074, -38.0573) knots 0 0 0 0 0.038666 0.078697 0.078697 0.078697 0.078697
  spline S1023 degree 3 poles (22.575, -137.0341) (22.5715, -137.3816) (22.5658, -137.949) (22.7801, -138.4707) (22.8632, -138.6729) knots 0 0 0 0 0.102785 0.167831 0.167831 0.167831 0.167831
  spline S1024 degree 3 poles (22.8632, -138.6729) (22.9611, -138.7917) (23.1477, -139.0182) (23.4369, -139.0604) (23.5743, -139.0805) knots 0 0 0 0 0.04439 0.084625 0.084625 0.084625 0.084625
  spline S1025 degree 3 poles (23.5743, -139.0805) (23.7118, -139.0603) (24.0013, -139.0177) (24.1876, -138.7905) (24.2855, -138.6712) knots 0 0 0 0 0.040246 0.084724 0.084724 0.084724 0.084724
  spline S1026 degree 3 poles (24.2855, -138.6712) (24.3685, -138.4689) (24.5825, -137.9476) (24.577, -137.3809) (24.5737, -137.0341) knots 0 0 0 0 0.065086 0.167658 0.167658 0.167658 0.167658
  spline S1027 degree 3 poles (24.5737, -137.0341) (24.5773, -136.6859) (24.5832, -136.1179) (24.3685, -135.5957) (24.2855, -135.3936) knots 0 0 0 0 0.102998 0.168003 0.168003 0.168003 0.168003
  spline S1028 degree 3 poles (24.2855, -135.3936) (24.1869, -135.2753) (23.9979, -135.0485) (23.7068, -135.0074) (23.5675, -134.9877) knots 0 0 0 0 0.044426 0.085146 0.085146 0.085146 0.085146
  spline S1029 degree 3 poles (23.5675, -134.9877) (23.4332, -135.0033) (23.1618, -135.0347) (22.9827, -135.2414) (22.8922, -135.3458) knots 0 0 0 0 0.039068 0.078965 0.078965 0.078965 0.078965
  spline S1030 degree 3 poles (22.8922, -135.3458) (22.8006, -135.56) (22.5713, -136.096) (22.5736, -136.6822) (22.575, -137.0341) knots 0 0 0 0 0.069271 0.173342 0.173342 0.173342 0.173342
  spline S1031 degree 3 poles (18.7722, -187.8799) (18.7778, -187.9846) (18.7892, -188.1944) (18.8676, -188.3894) (18.9069, -188.487) knots 0 0 0 0 0.031219 0.062565 0.062565 0.062565 0.062565
  spline S1032 degree 3 poles (18.9069, -188.487) (18.955, -188.5771) (19.0485, -188.752) (19.2069, -188.871) (19.2838, -188.9287) knots 0 0 0 0 0.03022 0.058691 0.058691 0.058691 0.058691
  spline S1033 degree 3 poles (19.2838, -188.9287) (19.3646, -188.973) (19.5233, -189.0599) (19.7035, -189.0737) (19.792, -189.0805) knots 0 0 0 0 0.027299 0.05358 0.05358 0.05358 0.05358
  spline S1034 degree 3 poles (19.792, -189.0805) (19.918, -189.0663) (20.1758, -189.0372) (20.3642, -188.8582) (20.4604, -188.7667) knots 0 0 0 0 0.036994 0.075673 0.075673 0.075673 0.075673
  spline S1035 degree 3 poles (20.4604, -188.7667) (20.5419, -188.6473) (20.7168, -188.391) (20.732, -188.0801) (20.7401, -187.9141) knots 0 0 0 0 0.042537 0.091301 0.091301 0.091301 0.091301
  spline S1036 degree 3 poles (20.7401, -187.9141) (20.732, -187.7543) (20.7169, -187.4549) (20.5443, -187.211) (20.4639, -187.0972) knots 0 0 0 0 0.046854 0.087822 0.087822 0.087822 0.087822
  spline S1037 degree 3 poles (20.4639, -187.0972) (20.3652, -187.0102) (20.1661, -186.8345) (19.9015, -186.8108) (19.7681, -186.7988) knots 0 0 0 0 0.038404 0.077492 0.077492 0.077492 0.077492
  spline S1038 degree 3 poles (19.7681, -186.7988) (19.6346, -186.8112) (19.3678, -186.8361) (19.164, -187.0102) (19.0621, -187.0972) knots 0 0 0 0 0.039172 0.078342 0.078342 0.078342 0.078342
  spline S1039 degree 3 poles (19.0621, -187.0972) (18.9776, -187.2076) (18.8011, -187.4381) (18.7821, -187.7286) (18.7722, -187.8799) knots 0 0 0 0 0.040772 0.085151 0.085151 0.085151 0.085151
  spline S1040 degree 3 poles (18.7718, -237.88) (18.7775, -237.9847) (18.7888, -238.1945) (18.8673, -238.3894) (18.9066, -238.4871) knots 0 0 0 0 0.031219 0.062565 0.062565 0.062565 0.062565
  spline S1041 degree 3 poles (18.9066, -238.4871) (18.9547, -238.5771) (19.0481, -238.7521) (19.2066, -238.871) (19.2834, -238.9287) knots 0 0 0 0 0.03022 0.058691 0.058691 0.058691 0.058691
  spline S1042 degree 3 poles (19.2834, -238.9287) (19.3643, -238.973) (19.5229, -239.0599) (19.7032, -239.0737) (19.7916, -239.0805) knots 0 0 0 0 0.027299 0.05358 0.05358 0.05358 0.05358
  spline S1043 degree 3 poles (19.7916, -239.0805) (19.9177, -239.0663) (20.1755, -239.0373) (20.3638, -238.8583) (20.4601, -238.7667) knots 0 0 0 0 0.036994 0.075673 0.075673 0.075673 0.075673
  spline S1044 degree 3 poles (20.4601, -238.7667) (20.5416, -238.6473) (20.7164, -238.3911) (20.7317, -238.0802) (20.7398, -237.9141) knots 0 0 0 0 0.042537 0.091301 0.091301 0.091301 0.091301
  spline S1045 degree 3 poles (20.7398, -237.9141) (20.7317, -237.7543) (20.7165, -237.4549) (20.544, -237.211) (20.4635, -237.0972) knots 0 0 0 0 0.046854 0.087822 0.087822 0.087822 0.087822
  spline S1046 degree 3 poles (20.4635, -237.0972) (20.3649, -237.0102) (20.1658, -236.8346) (19.9012, -236.8108) (19.7678, -236.7988) knots 0 0 0 0 0.038404 0.077492 0.077492 0.077492 0.077492
  spline S1047 degree 3 poles (19.7678, -236.7988) (19.6343, -236.8112) (19.3675, -236.8361) (19.1637, -237.0102) (19.0618, -237.0972) knots 0 0 0 0 0.039172 0.078342 0.078342 0.078342 0.078342
  spline S1048 degree 3 poles (19.0618, -237.0972) (18.9772, -237.2076) (18.8007, -237.4382) (18.7817, -237.7286) (18.7718, -237.88) knots 0 0 0 0 0.040772 0.085151 0.085151 0.085151 0.085151
  spline S1049 degree 3 poles (22.6088, -237.0342) (22.6053, -237.3816) (22.5996, -237.949) (22.8139, -238.4708) (22.897, -238.673) knots 0 0 0 0 0.102785 0.167831 0.167831 0.167831 0.167831
  spline S1050 degree 3 poles (22.897, -238.673) (22.9949, -238.7918) (23.1815, -239.0182) (23.4707, -239.0605) (23.6081, -239.0806) knots 0 0 0 0 0.04439 0.084625 0.084625 0.084625 0.084625
  spline S1051 degree 3 poles (23.6081, -239.0806) (23.7456, -239.0603) (24.0351, -239.0178) (24.2214, -238.7906) (24.3193, -238.6713) knots 0 0 0 0 0.040246 0.084724 0.084724 0.084724 0.084724
  spline S1052 degree 3 poles (24.3193, -238.6713) (24.4023, -238.4689) (24.6163, -237.9477) (24.6108, -237.3809) (24.6075, -237.0342) knots 0 0 0 0 0.065086 0.167658 0.167658 0.167658 0.167658
  spline S1053 degree 3 poles (24.6075, -237.0342) (24.6111, -236.686) (24.617, -236.118) (24.4023, -235.5957) (24.3193, -235.3937) knots 0 0 0 0 0.102998 0.168003 0.168003 0.168003 0.168003
  spline S1054 degree 3 poles (24.3193, -235.3937) (24.2207, -235.2753) (24.0317, -235.0486) (23.7406, -235.0075) (23.6013, -234.9878) knots 0 0 0 0 0.044426 0.085146 0.085146 0.085146 0.085146
  spline S1055 degree 3 poles (23.6013, -234.9878) (23.467, -235.0033) (23.1956, -235.0347) (23.0165, -235.2414) (22.926, -235.3459) knots 0 0 0 0 0.039068 0.078965 0.078965 0.078965 0.078965
  spline S1056 degree 3 poles (22.926, -235.3459) (22.8344, -235.5601) (22.6051, -236.0961) (22.6074, -236.6822) (22.6088, -237.0342) knots 0 0 0 0 0.069271 0.173342 0.173342 0.173342 0.173342
  spline S1057 degree 3 poles (22.5969, -337.034) (22.5934, -337.3815) (22.5877, -337.9488) (22.8021, -338.4706) (22.8851, -338.6728) knots 0 0 0 0 0.102785 0.167831 0.167831 0.167831 0.167831
  spline S1058 degree 3 poles (22.8851, -338.6728) (22.983, -338.7916) (23.1697, -339.018) (23.4588, -339.0603) (23.5963, -339.0803) knots 0 0 0 0 0.04439 0.084625 0.084625 0.084625 0.084625
  spline S1059 degree 3 poles (23.5963, -339.0803) (23.7338, -339.0601) (24.0232, -339.0176) (24.2096, -338.7903) (24.3074, -338.671) knots 0 0 0 0 0.040246 0.084724 0.084724 0.084724 0.084724
  spline S1060 degree 3 poles (24.3074, -338.671) (24.3904, -338.4687) (24.6044, -337.9474) (24.5989, -337.3807) (24.5955, -337.0339) knots 0 0 0 0 0.065086 0.167658 0.167658 0.167658 0.167658
  spline S1061 degree 3 poles (24.5955, -337.0339) (24.5991, -336.6857) (24.605, -336.1177) (24.3903, -335.5955) (24.3073, -335.3934) knots 0 0 0 0 0.102998 0.168003 0.168003 0.168003 0.168003
  spline S1062 degree 3 poles (24.3073, -335.3934) (24.2087, -335.2751) (24.0197, -335.0484) (23.7286, -335.0072) (23.5893, -334.9876) knots 0 0 0 0 0.044426 0.085146 0.085146 0.085146 0.085146
  spline S1063 degree 3 poles (23.5893, -334.9876) (23.455, -335.0031) (23.1836, -335.0345) (23.0045, -335.2413) (22.914, -335.3457) knots 0 0 0 0 0.039068 0.078965 0.078965 0.078965 0.078965
  spline S1064 degree 3 poles (22.914, -335.3457) (22.8224, -335.5599) (22.5931, -336.0959) (22.5955, -336.6821) (22.5969, -337.034) knots 0 0 0 0 0.069271 0.173342 0.173342 0.173342 0.173342
  line L685 (20.1493, -387.7401) -> (20.1493, -385.4856)
  line L686 (20.1493, -385.4856) -> (18.5839, -387.7401)
  line L687 (18.5839, -387.7401) -> (20.1493, -387.7401)
  line L688 (20.154, -437.7399) -> (20.1538, -435.4855)
  line L689 (20.1538, -435.4855) -> (18.5885, -437.74)
  line L690 (18.5885, -437.74) -> (20.154, -437.7399)
  spline S1065 degree 3 poles (22.7017, -437.0337) (22.6982, -437.3812) (22.6925, -437.9485) (22.9069, -438.4703) (22.99, -438.6725) knots 0 0 0 0 0.102785 0.167831 0.167831 0.167831 0.167831
  spline S1066 degree 3 poles (22.99, -438.6725) (23.0879, -438.7913) (23.2745, -439.0177) (23.5637, -439.0599) (23.7011, -439.08) knots 0 0 0 0 0.04439 0.084625 0.084625 0.084625 0.084625
  spline S1067 degree 3 poles (23.7011, -439.08) (23.8386, -439.0598) (24.1281, -439.0172) (24.3144, -438.79) (24.4122, -438.6707) knots 0 0 0 0 0.040246 0.084724 0.084724 0.084724 0.084724
  spline S1068 degree 3 poles (24.4122, -438.6707) (24.4953, -438.4683) (24.7092, -437.947) (24.7037, -437.3803) (24.7003, -437.0335) knots 0 0 0 0 0.065086 0.167658 0.167658 0.167658 0.167658
  spline S1069 degree 3 poles (24.7003, -437.0335) (24.7039, -436.6853) (24.7097, -436.1173) (24.495, -435.5951) (24.412, -435.393) knots 0 0 0 0 0.102998 0.168003 0.168003 0.168003 0.168003
  spline S1070 degree 3 poles (24.412, -435.393) (24.3134, -435.2747) (24.1244, -435.048) (23.8332, -435.0069) (23.694, -434.9872) knots 0 0 0 0 0.044426 0.085146 0.085146 0.085146 0.085146
  spline S1071 degree 3 poles (23.694, -434.9872) (23.5597, -435.0028) (23.2883, -435.0342) (23.1092, -435.2409) (23.0187, -435.3454) knots 0 0 0 0 0.039068 0.078965 0.078965 0.078965 0.078965
  spline S1072 degree 3 poles (23.0187, -435.3454) (22.9271, -435.5596) (22.6979, -436.0956) (22.7002, -436.6818) (22.7017, -437.0337) knots 0 0 0 0 0.069271 0.173342 0.173342 0.173342 0.173342
  spline S1073 degree 3 poles (22.6014, -537.0337) (22.5979, -537.3811) (22.5923, -537.9485) (22.8067, -538.4702) (22.8897, -538.6724) knots 0 0 0 0 0.102785 0.167831 0.167831 0.167831 0.167831
  spline S1074 degree 3 poles (22.8897, -538.6724) (22.9876, -538.7912) (23.1743, -539.0177) (23.4634, -539.0599) (23.6009, -539.08) knots 0 0 0 0 0.04439 0.084625 0.084625 0.084625 0.084625
  spline S1075 degree 3 poles (23.6009, -539.08) (23.7384, -539.0597) (24.0279, -539.0171) (24.2142, -538.7899) (24.312, -538.6706) knots 0 0 0 0 0.040246 0.084724 0.084724 0.084724 0.084724
  spline S1076 degree 3 poles (24.312, -538.6706) (24.395, -538.4683) (24.609, -537.947) (24.6034, -537.3802) (24.6, -537.0335) knots 0 0 0 0 0.065086 0.167658 0.167658 0.167658 0.167658
  spline S1077 degree 3 poles (24.6, -537.0335) (24.6036, -536.6853) (24.6095, -536.1173) (24.3948, -535.5951) (24.3117, -535.393) knots 0 0 0 0 0.102998 0.168003 0.168003 0.168003 0.168003
  spline S1078 degree 3 poles (24.3117, -535.393) (24.2131, -535.2747) (24.0241, -535.048) (23.733, -535.0068) (23.5937, -534.9872) knots 0 0 0 0 0.044426 0.085146 0.085146 0.085146 0.085146
  spline S1079 degree 3 poles (23.5937, -534.9872) (23.4594, -535.0027) (23.188, -535.0342) (23.0089, -535.2409) (22.9184, -535.3454) knots 0 0 0 0 0.039068 0.078965 0.078965 0.078965 0.078965
  spline S1080 degree 3 poles (22.9184, -535.3454) (22.8268, -535.5596) (22.5976, -536.0956) (22.6, -536.6817) (22.6014, -537.0337) knots 0 0 0 0 0.069271 0.173342 0.173342 0.173342 0.173342
  spline S1081 degree 3 poles (22.641, -637.0339) (22.6375, -637.3814) (22.6319, -637.9488) (22.8462, -638.4705) (22.9293, -638.6728) knots 0 0 0 0 0.102785 0.167831 0.167831 0.167831 0.167831
  spline S1082 degree 3 poles (22.9293, -638.6728) (23.0272, -638.7915) (23.2138, -639.018) (23.5029, -639.0602) (23.6404, -639.0803) knots 0 0 0 0 0.04439 0.084625 0.084625 0.084625 0.084625
  spline S1083 degree 3 poles (23.6404, -639.0803) (23.7779, -639.0601) (24.0674, -639.0175) (24.2537, -638.7903) (24.3515, -638.671) knots 0 0 0 0 0.040246 0.084724 0.084724 0.084724 0.084724
  spline S1084 degree 3 poles (24.3515, -638.671) (24.4346, -638.4687) (24.6486, -637.9474) (24.643, -637.3806) (24.6397, -637.0339) knots 0 0 0 0 0.065086 0.167658 0.167658 0.167658 0.167658
  spline S1085 degree 3 poles (24.6397, -637.0339) (24.6433, -636.6857) (24.6492, -636.1177) (24.4345, -635.5955) (24.3514, -635.3934) knots 0 0 0 0 0.102998 0.168003 0.168003 0.168003 0.168003
  spline S1086 degree 3 poles (24.3514, -635.3934) (24.2528, -635.2751) (24.0639, -635.0483) (23.7727, -635.0072) (23.6335, -634.9875) knots 0 0 0 0 0.044426 0.085146 0.085146 0.085146 0.085146
  spline S1087 degree 3 poles (23.6335, -634.9875) (23.4992, -635.0031) (23.2277, -635.0345) (23.0487, -635.2412) (22.9582, -635.3457) knots 0 0 0 0 0.039068 0.078965 0.078965 0.078965 0.078965
  spline S1088 degree 3 poles (22.9582, -635.3457) (22.8666, -635.5599) (22.6373, -636.0959) (22.6396, -636.682) (22.641, -637.0339) knots 0 0 0 0 0.069271 0.173342 0.173342 0.173342 0.173342
  spline S1089 degree 3 poles (22.363, -737.034) (22.3595, -737.3815) (22.3539, -737.9488) (22.5682, -738.4706) (22.6513, -738.6728) knots 0 0 0 0 0.102785 0.167831 0.167831 0.167831 0.167831
  spline S1090 degree 3 poles (22.6513, -738.6728) (22.7492, -738.7916) (22.9358, -739.018) (23.2249, -739.0603) (23.3624, -739.0803) knots 0 0 0 0 0.04439 0.084625 0.084625 0.084625 0.084625
  spline S1091 degree 3 poles (23.3624, -739.0803) (23.4999, -739.0601) (23.7894, -739.0175) (23.9757, -738.7903) (24.0735, -738.671) knots 0 0 0 0 0.040246 0.084724 0.084724 0.084724 0.084724
  spline S1092 degree 3 poles (24.0735, -738.671) (24.1566, -738.4687) (24.3706, -737.9474) (24.365, -737.3807) (24.3617, -737.0339) knots 0 0 0 0 0.065086 0.167658 0.167658 0.167658 0.167658
  spline S1093 degree 3 poles (24.3617, -737.0339) (24.3653, -736.6857) (24.3712, -736.1177) (24.1565, -735.5955) (24.0734, -735.3934) knots 0 0 0 0 0.102998 0.168003 0.168003 0.168003 0.168003
  spline S1094 degree 3 poles (24.0734, -735.3934) (23.9748, -735.2751) (23.7859, -735.0484) (23.4947, -735.0072) (23.3555, -734.9876) knots 0 0 0 0 0.044426 0.085146 0.085146 0.085146 0.085146
  spline S1095 degree 3 poles (23.3555, -734.9876) (23.2212, -735.0031) (22.9497, -735.0345) (22.7707, -735.2412) (22.6802, -735.3457) knots 0 0 0 0 0.039068 0.078965 0.078965 0.078965 0.078965
  spline S1096 degree 3 poles (22.6802, -735.3457) (22.5886, -735.5599) (22.3593, -736.0959) (22.3616, -736.682) (22.363, -737.034) knots 0 0 0 0 0.069271 0.173342 0.173342 0.173342 0.173342
  spline S1097 degree 3 poles (19.6875, -837.034) (19.684, -837.3815) (19.6783, -837.9489) (19.8927, -838.4706) (19.9758, -838.6728) knots 0 0 0 0 0.102785 0.167831 0.167831 0.167831 0.167831
  spline S1098 degree 3 poles (19.9758, -838.6728) (20.0736, -838.7916) (20.2603, -839.0181) (20.5494, -839.0603) (20.6869, -839.0804) knots 0 0 0 0 0.04439 0.084625 0.084625 0.084625 0.084625
  spline S1099 degree 3 poles (20.6869, -839.0804) (20.8244, -839.0601) (21.1139, -839.0176) (21.3002, -838.7903) (21.398, -838.6711) knots 0 0 0 0 0.040246 0.084724 0.084724 0.084724 0.084724
  spline S1100 degree 3 poles (21.398, -838.6711) (21.4811, -838.4687) (21.695, -837.9474) (21.6895, -837.3807) (21.6861, -837.0339) knots 0 0 0 0 0.065086 0.167658 0.167658 0.167658 0.167658
  spline S1101 degree 3 poles (21.6861, -837.0339) (21.6897, -836.6857) (21.6956, -836.1177) (21.4809, -835.5955) (21.3979, -835.3934) knots 0 0 0 0 0.102998 0.168003 0.168003 0.168003 0.168003
  spline S1102 degree 3 poles (21.3979, -835.3934) (21.2993, -835.2751) (21.1103, -835.0484) (20.8192, -835.0073) (20.6799, -834.9876) knots 0 0 0 0 0.044426 0.085146 0.085146 0.085146 0.085146
  spline S1103 degree 3 poles (20.6799, -834.9876) (20.5456, -835.0031) (20.2742, -835.0346) (20.0951, -835.2413) (20.0046, -835.3457) knots 0 0 0 0 0.039068 0.078965 0.078965 0.078965 0.078965